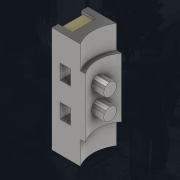
# Autodesk Inventor part: Button
Saved by Autodesk Inventor 2021 (Build 250183000, 183)
## iProperties
Created: 2021-01-08
Part Number: Button
Material: Generic
Document SubType Name: Modeling
Designer: Alex
Density: 1 g/cm^3
Appearance: Default
Author: Alex
Autodesk Inventor part; units mm, degrees
sketch "Sketch1" plane through (0, 0, 0) normal (0, 1, 0) x (-1, 0, 0)
  circle A0 centre (0, 0) radius 14
  line L0 (14, 0) -> (27, 0)
  circle A1 centre (0, 0) radius 16
  line L1 (27, 0) -> (27, -8.5)
  line L2 (27, -8.5) -> (13.5552, -8.5)
  line L3 (13.5552, 8.5) -> (27, 8.5)
  line L4 (27, 8.5) -> (27, -8.5)
  line L5 (13.5552, 8.5) -> (11.1243, 8.5)
  line L6 (13.5552, -8.5) -> (11.1243, -8.5)
  line L7 (13.5552, 8.5) -> (13.5552, -8.5)
  dimension "d0" = 28
  dimension "d1" = 13
  dimension "d2" = 32
  dimension "d3" = 8.5
  dimension "d5" = 17
  constraints: 16 end point, 4 horizontal, 3 point on circle, 2 centre point, 2 coincident, 2 vertical, 1 parallel
  measures "d0" diameter of A0
  measures "d1" distance of L0.start L0.end
  measures "d2" diameter of A1
  measures "d3" distance of L0.end L1.end
  measures "d5" distance of L2.end L3.start
extrude "Extrusion1" add sketch "Sketch1" along normal blind 50 contours L5 L7 A0 | A0 L7 L6 | L7 A1 L0 A0 | L3 L4 L0 A1 | A0 L0 A1 L7 | A1 L0 L1 L2
ref_plane "Work Plane1" through (0, 11, 0) normal (0, -1, 0) x (1, 0, 0)
sketch "Sketch2" plane through (0, 11, 0) normal (0, -1, 0) x (1, 0, 0)
  circle A0 centre (0, 0) radius 16
  line L0 (-11.1243, -8.5) -> (-27, -8.5) projected
  circle A1 centre (0, 0) radius 14
  line L1 (-27, 8.5) -> (-11.1243, 8.5) projected
  line L2 (-13.5554, 8.5) -> (-11.1243, 8.5)
  line L3 (-13.5554, -8.5) -> (-11.1243, -8.5)
  dimension "d9" = 32
  constraints: 4 end point, 3 point on circle, 2 centre point, 2 coincident, 2 point on line, 1 collinear, 1 horizontal
  measures "d9" diameter of A0
extrude "Extrusion2" cut sketch "Sketch2" against normal blind 28 contours L1 A1 L0 A0 picked at (-13.7856, -6.5585)
ref_plane "Work Plane2" through (-13.5554, 11, 8.5) normal (-1, 0, 0) x (0, 1, 0)
sketch "Sketch3" plane through (-13.5554, 11, 8.5) normal (-1, 0, 0) x (0, 1, 0)
  line L0 (28, 17) -> (28, 0) construction
  line L1 (28, 8.5) -> (0, 8.5) construction
  line L2 (0, 17) -> (0, 0) construction
  line L3 (28, 8.5) -> (19, 8.5)
  circle A0 centre (19, 8.5) radius 3
  line L4 (0, 8.5) -> (9, 8.5)
  circle A1 centre (9, 8.5) radius 3
  point P0 (-11, 8.5)
  dimension "d14" = 9
  dimension "d15" = 6
  dimension "d17" = 9
  dimension "d18" = 6
  constraints: 6 end point, 2 centre point, 2 coincident, 2 midpoint, 2 point on line
  measures "d14" distance of L1.start L3.end
  measures "d15" diameter of A0
  measures "d17" distance of L1.end L4.end
  measures "d18" diameter of A1
extrude "Extrusion3" add sketch "Sketch3" along normal up to surface
sketch "Sketch4" plane through (-13.5554, 30, 0) normal (1, 0, 0) x (0, 0, -1)
  circle A0 centre (0, 0) radius 3 projected
  circle A1 centre (0, 0) radius 3
  point P0 (0, -30)
  constraints: 1 centre point, 1 coincident
sketch "Sketch5" plane through (-13.5554, 20, 0) normal (1, 0, 0) x (0, 0, -1)
  circle A0 centre (0, 0) radius 3
  point P0 (0, -20)
  constraints: 1 centre point
extrude "Extrusion4" cut sketch "Sketch4" against normal blind 0.445
extrude "Extrusion5" cut sketch "Sketch5" against normal blind 0.445
sketch "Sketch6" plane through (-14.0004, 30, 0) normal (1, 0, 0) x (0, 0, -1)
  circle A0 centre (0, 0) radius 3
  point P0 (0, -30)
  constraints: 1 centre point
sketch "Sketch7" plane through (-14.0004, 20, 0) normal (1, 0, 0) x (0, 0, -1)
  circle A0 centre (0, 0) radius 3
  point P0 (0, -20)
  constraints: 1 centre point
extrude "Extrusion6" add sketch "Sketch6" along normal blind 6
extrude "Extrusion7" add sketch "Sketch7" along normal up to surface (6 mm away)
sketch "Sketch8" plane through (0, 11, 0) normal (0, 1, 0) x (1, 0, 0)
  circle A0 centre (0, 0) radius 14
  circle A1 centre (0, 0) radius 16
  line L0 (-13.5554, 8.5) -> (-11.1243, 8.5) projected
  line L1 (-13.5554, 8.5) -> (-11.1243, 8.5)
  arc A2 (-11.1243, 8.5) -> (-11.1243, -8.5) centre (0, 0) ccw projected
  line L2 (-13.5554, -8.5) -> (-11.1243, -8.5)
  dimension "d29" = 32
  constraints: 4 end point, 2 centre point, 2 coincident, 1 collinear, 1 horizontal
  measures "d29" diameter of A1
sketch "Sketch9" plane through (0, 11, 0) normal (0, 1, 0) x (1, 0, 0)
  circle A0 centre (0, 0) radius 16
  circle A1 centre (0, 0) radius 14
  dimension "d30" = 32
  constraints: 2 centre point, 2 coincident
  measures "d30" diameter of A0
extrude "Extrusion8" add sketch "Sketch8" along normal up to surface (28 mm away) contours A0 L2 A1 L0 picked at (-13.7856, -6.5585)
extrude "Extrusion9" cut sketch "Sketch9" against normal up to surface (11 mm away)
ref_plane "Work Plane3" through (0, 39, 0) normal (0, 1, 0) x (1, 0, 0)
sketch "Sketch10" plane through (0, 39, 0) normal (0, 1, 0) x (1, 0, 0)
  circle A0 centre (0, 0) radius 16
  circle A1 centre (0, 0) radius 14
  dimension "d36" = 32
  dimension "d37" = 28
  constraints: 2 centre point, 2 coincident
  measures "d36" diameter of A0
  measures "d37" diameter of A1
extrude "Extrusion10" cut sketch "Sketch10" along normal up to surface (11 mm away)
sketch "Sketch11" plane through (-27, 0, -8.5) normal (-1, 0, 0) x (0, 0, 1)
  line L0 (17, 0) -> (17, 50) projected
  line L1 (17, 50) -> (14, 50)
  line L2 (0, 50) -> (17, 50) projected
  line L3 (14, 50) -> (3, 50)
  line L4 (0, 0) -> (0, 50) projected
  line L5 (0, 0) -> (3, 0)
  line L6 (17, 0) -> (0, 0) projected
  line L7 (14, 50) -> (3, 50)
  line L8 (3, 50) -> (3, 0)
  line L9 (3, 0) -> (14, 0)
  line L10 (14, 0) -> (14, 50)
  point P0 (8.5, 0)
  dimension "d40" = 3
  dimension "d41" = 11
  dimension "d42" = 3
  constraints: 14 end point, 3 point on line, 2 parallel, 1 horizontal, 1 perpendicular
  measures "d40" distance of L0.end L1.end
  measures "d41" distance of L1.end L3.end
  measures "d42" distance of L4.start L5.end
extrude "Extrusion11" cut sketch "Sketch11" against normal blind 1 contours L6 L8 L2 L10
sketch "Sketch12" plane through (0, 50, 0) normal (0, 1, 0) x (1, 0, 0)
  line L0 (-27, -5.5) -> (-27, -8.5) projected
  line L1 (-27, -5.5) -> (-20.278, -5.5)
  line L2 (-27, 5.5) -> (-26, 5.5) projected
  line L3 (-20.278, -5.5) -> (-27, -5.5)
  line L4 (-27, -5.5) -> (-27, 5.5)
  line L5 (-27, 5.5) -> (-20.278, 5.5)
  line L6 (-20.278, 5.5) -> (-20.278, -5.5)
  point P0 (0, 0)
  dimension "d45" = 6.722
  constraints: 10 end point, 2 horizontal, 2 parallel, 1 perpendicular
  measures "d45" distance of L0.start L1.end
sketch "Sketch13" plane through (0, 0, 0) normal (0, -1, 0) x (1, 0, 0)
  line L0 (-27, -5.5) -> (-26, -5.5) projected
  line L1 (-27, -5.5) -> (-20.278, -5.5)
  line L2 (-20.278, -5.5) -> (-27, -5.5)
  line L3 (-27, -5.5) -> (-27, 5.5)
  line L4 (-27, 5.5) -> (-20.278, 5.5)
  line L5 (-20.278, 5.5) -> (-20.278, -5.5)
  point P0 (0, 0)
  dimension "d46" = 6.722
  constraints: 10 end point, 2 horizontal, 2 parallel, 1 perpendicular
  measures "d46" distance of L0.start L1.end
extrude "Extrusion12" cut sketch "Sketch13" against normal blind 1
extrude "Extrusion13" cut sketch "Sketch12" against normal blind 1
sketch "Sketch14" plane through (-27, 0, 8.5) normal (0, 0, 1) x (1, 0, 0)
  line L0 (0, 50) -> (6.722, 50) construction
  line L1 (6.722, 50) -> (6.722, 41) construction
  line L2 (6.722, 41) -> (6.722, 34) construction
  line L3 (0, 34) -> (0, 31) construction
  line L4 (0, 31) -> (3.361, 31) construction
  line L5 (6.722, 34) -> (3.361, 34) construction
  line L6 (3.361, 34) -> (3.361, 31) construction
  line L7 (3.361, 31) -> (4.861, 31) construction
  line L8 (0, 0) -> (0, 50) construction
  line L9 (4.861, 31) -> (4.861, 38.2796) construction
  line L10 (4.861, 31) -> (7.861, 31) construction
  line L11 (13, 39) -> (13, 11) construction
  line L12 (6.361, 31) -> (6.361, 37.5) construction
  line L13 (4.861, 36.5) -> (7.861, 36.5) construction
  line L14 (7.861, 36.5) -> (7.861, 31.5) construction
  line L15 (7.861, 31.5) -> (4.861, 31.5) construction
  line L16 (4.861, 31.5) -> (4.861, 36.5) construction
  line L17 (4.861, 36.5) -> (7.861, 31.5) construction
  line L18 (7.861, 36.5) -> (4.861, 31.5) construction
  line L19 (6.361, 31.5) -> (6.361, 20.5) construction
  line L20 (6.361, 20.5) -> (6.361, 18) construction
  line L21 (4.861, 15.5) -> (7.861, 15.5) construction
  line L22 (7.861, 15.5) -> (7.861, 20.5) construction
  line L23 (7.861, 20.5) -> (4.861, 20.5) construction
  line L24 (4.861, 20.5) -> (4.861, 15.5) construction
  line L25 (4.861, 15.5) -> (7.861, 20.5) construction
  line L26 (7.861, 15.5) -> (4.861, 20.5) construction
  line L27 (8.861, 21.5) -> (8.861, 14.5)
  line L28 (8.861, 14.5) -> (3.861, 14.5)
  line L29 (3.861, 14.5) -> (3.861, 21.5)
  line L30 (3.861, 21.5) -> (8.861, 21.5)
  line L31 (8.861, 37.5) -> (3.861, 37.5)
  line L32 (3.861, 37.5) -> (3.861, 30.5)
  line L33 (3.861, 30.5) -> (8.861, 30.5)
  line L34 (8.861, 30.5) -> (8.861, 37.5)
  point P0 (27, 0)
  point P1 (6.361, 34)
  dimension "d51" = 9
  dimension "d52" = 7
  dimension "d53" = 3
  dimension "d54" = 1.5
  dimension "d55" = 3
  dimension "d56" = 3
  dimension "d57" = 5
  dimension "d58" = 11
  dimension "d59" = 2.5
  dimension "d60" = 1
  dimension "d61" = 1
  constraints: 64 end point, 9 parallel, 9 perpendicular, 6 midpoint, 4 point on line, 3 vertical, 2 horizontal, 6 other
  measures "d51" distance of L0.end L1.end
  measures "d52" distance of L1.end L2.end
  measures "d53" distance of L3.start L3.end
  measures "d54" distance of L4.end L7.end
  measures "d55" distance of L7.end L10.end
  measures "d56" distance of L14.end L15.end
  measures "d57" distance of L13.end L14.end
  measures "d58" distance of L19.start L19.end
  measures "d59" distance of L19.end L20.end
  measures "d60" distance between parallel lines of L22 L27
  measures "d61" distance between parallel lines of L13 L31
extrude "Extrusion14" cut sketch "Sketch14" against normal blind 5
body "Solid1"
